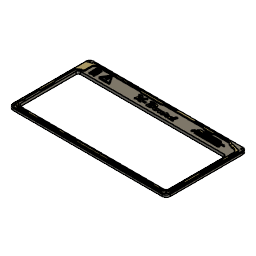
top (Autodesk Fusion 360 design; units mm, degrees)
part number: 2026-05-16-16-15-53-666
Autodesk Fusion 360 part; units mm, degrees
(part 1 of 5)
sketch "Sketch1" plane through (0, 0, 0) normal (0, 0, 1) x (1, 0, 0)
  line L0 (47.7197, -65.9177) -> (60.7197, -65.9177)
  line L1 (52.4822, -41.8177) -> (65.4822, -41.8177)
  line L2 (52.4822, -27.8177) -> (65.4822, -27.8177)
  arc A0 (170.2572, -3.7177) -> (170.7572, -3.2177) centre (170.2572, -3.2177) ccw
  line L3 (189.8072, 9.7823) -> (189.8072, -3.2177)
  arc A1 (180.2822, -9.2677) -> (179.7822, -8.7677) centre (179.7822, -9.2677) ccw
  line L4 (208.8572, 9.7823) -> (208.8572, -3.2177)
  arc A2 (208.8572, 9.7823) -> (208.3572, 10.2823) centre (208.3572, 9.7823) ccw
  arc A3 (195.3572, 10.2823) -> (194.8572, 9.7823) centre (195.3572, 9.7823) ccw
  arc A4 (182.2202, -9.7677) -> (181.7202, -10.2677) centre (182.2202, -10.2677) ccw
  arc A5 (208.3572, -3.7177) -> (208.8572, -3.2177) centre (208.3572, -3.2177) ccw
  line L5 (195.3572, 10.2823) -> (208.3572, 10.2823)
  line L6 (195.3572, -3.7177) -> (208.3572, -3.7177)
  line L7 (176.3072, -3.7177) -> (189.3072, -3.7177)
  line L8 (176.3072, 10.2823) -> (189.3072, 10.2823)
  arc A6 (175.8072, -3.2177) -> (176.3072, -3.7177) centre (176.3072, -3.2177) ccw
  arc A7 (195.3572, -8.7677) -> (194.8572, -9.2677) centre (195.3572, -9.2677) ccw
  arc A8 (176.3072, 10.2823) -> (175.8072, 9.7823) centre (176.3072, 9.7823) ccw
  line L9 (195.3572, -8.7677) -> (208.3572, -8.7677)
  arc A9 (170.7572, 9.7823) -> (170.2572, 10.2823) centre (170.2572, 9.7823) ccw
  arc A10 (177.9009, -47.3677) -> (177.4009, -46.8677) centre (177.4009, -47.3677) ccw
  arc A11 (208.8572, -28.3177) -> (208.3572, -27.8177) centre (208.3572, -28.3177) ccw
  arc A12 (171.5447, -27.8177) -> (171.0447, -28.3177) centre (171.5447, -28.3177) ccw
  line L10 (146.9447, -47.3677) -> (146.9447, -60.3677)
  arc A13 (188.2202, -24.7677) -> (188.7202, -24.2677) centre (188.2202, -24.2677) ccw
  line L11 (171.0447, -28.3177) -> (171.0447, -41.3177)
  line L12 (-5.4553, -47.3677) -> (-5.4553, -60.3677)
  arc A14 (195.3572, -27.8177) -> (194.8572, -28.3177) centre (195.3572, -28.3177) ccw
  arc A15 (162.4629, -48.3677) -> (161.9629, -47.8677) centre (161.9629, -48.3677) ccw
  line L13 (208.8572, -9.2677) -> (208.8572, -22.2677)
  line L14 (132.9447, -47.3677) -> (132.9447, -60.3677)
  arc A16 (195.3572, -46.8677) -> (194.8572, -47.3677) centre (195.3572, -47.3677) ccw
  line L15 (180.2822, -9.2677) -> (180.2822, -22.2677)
  arc A17 (186.3389, -48.3677) -> (185.8389, -47.8677) centre (185.8389, -48.3677) ccw
  line L16 (181.7202, -10.2677) -> (181.7202, -24.2677)
  line L17 (-24.5053, -47.3677) -> (-24.5053, -60.3677)
  line L18 (-113.7226, -118.8427) -> (-113.7226, 57.4273)
  line L19 (42.9572, 10.2823) -> (55.9572, 10.2823)
  line L20 (188.7202, -10.2677) -> (188.7202, -24.2677)
  arc A18 (37.4072, -9.2677) -> (36.9072, -8.7677) centre (36.9072, -9.2677) ccw
  line L21 (-43.5553, -47.3677) -> (-43.5553, -60.3677)
  line L22 (194.8572, -9.2677) -> (194.8572, -22.2677)
  line L23 (75.7947, -47.3677) -> (75.7947, -60.3677)
  line L24 (-57.5553, -47.3677) -> (-57.5553, -60.3677)
  line L25 (194.8572, -47.3677) -> (194.8572, -60.3677)
  line L26 (42.9572, -3.7177) -> (55.9572, -3.7177)
  line L27 (177.9009, -47.3677) -> (177.9009, -60.3677)
  arc A19 (55.9572, -3.7177) -> (56.4572, -3.2177) centre (55.9572, -3.2177) ccw
  arc A20 (56.4572, 9.7823) -> (55.9572, 10.2823) centre (55.9572, 9.7823) ccw
  arc A21 (17.8572, -3.7177) -> (18.3572, -3.2177) centre (17.8572, -3.2177) ccw
  line L28 (194.8572, 9.7823) -> (194.8572, -3.2177)
  arc A22 (194.8572, -3.2177) -> (195.3572, -3.7177) centre (195.3572, -3.2177) ccw
  line L29 (175.8072, 9.7823) -> (175.8072, -3.2177)
  arc A23 (188.7202, -10.2677) -> (188.2202, -9.7677) centre (188.2202, -10.2677) ccw
  arc A24 (208.8572, -47.3677) -> (208.3572, -46.8677) centre (208.3572, -47.3677) ccw
  line L30 (171.5447, -27.8177) -> (184.5447, -27.8177)
  arc A25 (179.7822, -22.7677) -> (180.2822, -22.2677) centre (179.7822, -22.2677) ccw
  line L31 (163.9009, -47.3677) -> (163.9009, -60.3677)
  line L32 (195.3572, -46.8677) -> (208.3572, -46.8677)
  line L33 (94.8447, -47.3677) -> (94.8447, -60.3677)
  line L34 (182.2202, -24.7677) -> (188.2202, -24.7677)
  line L35 (179.8389, -47.8677) -> (185.8389, -47.8677)
  line L36 (208.8572, -28.3177) -> (208.8572, -41.3177)
  arc A26 (184.5447, -41.8177) -> (185.0447, -41.3177) centre (184.5447, -41.3177) ccw
  arc A27 (185.0447, -28.3177) -> (184.5447, -27.8177) centre (184.5447, -28.3177) ccw
  arc A28 (189.3072, -3.7177) -> (189.8072, -3.2177) centre (189.3072, -3.2177) ccw
  arc A29 (189.8072, 9.7823) -> (189.3072, 10.2823) centre (189.3072, 9.7823) ccw
  line L37 (182.2202, -9.7677) -> (188.2202, -9.7677)
  line L38 (47.7197, -79.9177) -> (60.7197, -79.9177)
  line L39 (57.2447, -46.8677) -> (70.2447, -46.8677)
  line L40 (-113.7226, 57.4273) -> (228.9474, 57.4273)
  line L41 (18.6447, -47.3677) -> (18.6447, -60.3677)
  line L42 (89.7947, -47.3677) -> (89.7947, -60.3677)
  arc A30 (36.9072, -3.7177) -> (37.4072, -3.2177) centre (36.9072, -3.2177) ccw
  arc A31 (42.9572, -8.7677) -> (42.4572, -9.2677) centre (42.9572, -9.2677) ccw
  line L43 (56.7447, -47.3677) -> (56.7447, -60.3677)
  line L44 (51.6947, -47.3677) -> (51.6947, -60.3677)
  line L45 (-0.4053, -47.3677) -> (-0.4053, -60.3677)
  line L46 (208.8572, -47.3677) -> (208.8572, -60.3677)
  arc A32 (37.4072, 9.7823) -> (36.9072, 10.2823) centre (36.9072, 9.7823) ccw
  line L47 (13.5947, -47.3677) -> (13.5947, -60.3677)
  line L48 (-83.7491, -47.3677) -> (-83.7491, -60.3677)
  line L49 (-38.5053, -47.3677) -> (-38.5053, -60.3677)
  line L50 (127.8947, -47.3677) -> (127.8947, -60.3677)
  line L51 (37.6947, -47.3677) -> (37.6947, -60.3677)
  arc A33 (23.9072, -8.7677) -> (23.4072, -9.2677) centre (23.9072, -9.2677) ccw
  arc A34 (179.8389, -47.8677) -> (179.3389, -48.3677) centre (179.8389, -48.3677) ccw
  line L52 (70.7447, -47.3677) -> (70.7447, -60.3677)
  line L53 (-19.4553, -47.3677) -> (-19.4553, -60.3677)
  arc A35 (56.4572, -9.2677) -> (55.9572, -8.7677) centre (55.9572, -9.2677) ccw
  line L54 (113.8947, -47.3677) -> (113.8947, -60.3677)
  arc A36 (23.9072, 10.2823) -> (23.4072, 9.7823) centre (23.9072, 9.7823) ccw
  line L55 (108.8447, -47.3677) -> (108.8447, -60.3677)
  line L56 (-69.7491, -47.3677) -> (-69.7491, -60.3677)
  line L57 (32.6447, -47.3677) -> (32.6447, -60.3677)
  line L58 (-18.9553, -60.8677) -> (-5.9553, -60.8677)
  line L59 (-23.7178, -27.8177) -> (-10.7178, -27.8177)
  line L60 (228.9474, 57.4273) -> (228.9474, -118.8427)
  arc A37 (18.3572, -9.2677) -> (17.8572, -8.7677) centre (17.8572, -9.2677) ccw
  line L61 (-28.4803, -65.9177) -> (-15.4803, -65.9177)
  line L62 (-33.2428, 10.2823) -> (-20.2428, 10.2823)
  arc A38 (42.4572, -3.2177) -> (42.9572, -3.7177) centre (42.9572, -3.2177) ccw
  line L63 (23.9072, -8.7677) -> (36.9072, -8.7677)
  line L64 (-33.2428, -8.7677) -> (-20.2428, -8.7677)
  line L65 (42.4572, 9.7823) -> (42.4572, -3.2177)
  line L66 (-23.7178, -41.8177) -> (-10.7178, -41.8177)
  line L67 (18.3572, 9.7823) -> (18.3572, -3.2177)
  line L68 (119.1572, -8.7677) -> (132.1572, -8.7677)
  arc A39 (155.9629, -47.8677) -> (155.4629, -48.3677) centre (155.9629, -48.3677) ccw
  line L69 (-28.4803, -79.9177) -> (-15.4803, -79.9177)
  line L70 (123.9197, -79.9177) -> (136.9197, -79.9177)
  line L71 (-57.0553, -60.8677) -> (-44.0553, -60.8677)
  line L72 (128.6822, -27.8177) -> (141.6822, -27.8177)
  line L73 (-64.1991, -98.9677) -> (-51.1991, -98.9677)
  line L74 (-64.1991, -84.9677) -> (-51.1991, -84.9677)
  line L75 (128.6822, -41.8177) -> (141.6822, -41.8177)
  line L76 (42.9572, -8.7677) -> (55.9572, -8.7677)
  line L77 (9.6197, -79.9177) -> (22.6197, -79.9177)
  line L78 (19.1447, -60.8677) -> (32.1447, -60.8677)
  line L79 (-33.2428, -22.7677) -> (-20.2428, -22.7677)
  line L80 (133.4447, -60.8677) -> (146.4447, -60.8677)
  arc A40 (157.2572, 10.2823) -> (156.7572, 9.7823) centre (157.2572, 9.7823) ccw
  line L81 (123.9197, -65.9177) -> (136.9197, -65.9177)
  line L82 (9.6197, -65.9177) -> (22.6197, -65.9177)
  line L83 (119.1572, -22.7677) -> (132.1572, -22.7677)
  line L84 (119.1572, -3.7177) -> (132.1572, -3.7177)
  line L85 (28.6697, -79.9177) -> (41.6697, -79.9177)
  line L86 (119.1572, 10.2823) -> (132.1572, 10.2823)
  line L87 (85.8197, -65.9177) -> (98.8197, -65.9177)
  line L88 (37.4072, 9.7823) -> (37.4072, -3.2177)
  line L89 (138.2072, -8.7677) -> (151.2072, -8.7677)
  line L90 (4.8572, -8.7677) -> (17.8572, -8.7677)
  line L91 (-9.4303, -79.9177) -> (3.5697, -79.9177)
  line L92 (-9.9303, -66.4177) -> (-9.9303, -79.4177)
  arc A41 (-44.0553, -60.8677) -> (-43.5553, -60.3677) centre (-44.0553, -60.3677) ccw
  line L93 (-78.9866, -66.4177) -> (-78.9866, -79.4177)
  line L94 (-15.4491, -85.9677) -> (-9.4491, -85.9677)
  line L95 (-86.9246, -66.9177) -> (-80.9246, -66.9177)
  arc A42 (132.6572, -9.2677) -> (132.1572, -8.7677) centre (132.1572, -9.2677) ccw
  arc A43 (85.8197, -65.9177) -> (85.3197, -66.4177) centre (85.8197, -66.4177) ccw
  arc A44 (-64.6991, -98.4677) -> (-64.1991, -98.9677) centre (-64.1991, -98.4677) ccw
  arc A45 (28.1697, -79.4177) -> (28.6697, -79.9177) centre (28.6697, -79.4177) ccw
  arc A46 (-56.5486, -67.4177) -> (-57.0486, -66.9177) centre (-57.0486, -67.4177) ccw
  arc A47 (56.7447, -60.3677) -> (57.2447, -60.8677) centre (57.2447, -60.3677) ccw
  line L96 (-71.3428, 10.2823) -> (-58.3428, 10.2823)
  line L97 (-9.4303, -65.9177) -> (3.5697, -65.9177)
  arc A48 (156.7572, -3.2177) -> (157.2572, -3.7177) centre (157.2572, -3.2177) ccw
  line L98 (4.8572, 10.2823) -> (17.8572, 10.2823)
  line L99 (31.0509, -84.9677) -> (44.0509, -84.9677)
  line L100 (-88.0116, -98.9677) -> (-75.0116, -98.9677)
  arc A49 (32.1447, -60.8677) -> (32.6447, -60.3677) centre (32.1447, -60.3677) ccw
  arc A50 (44.5509, -85.4677) -> (44.0509, -84.9677) centre (44.0509, -85.4677) ccw
  line L101 (56.4572, 9.7823) -> (56.4572, -3.2177)
  arc A51 (189.3072, -79.9177) -> (189.8072, -79.4177) centre (189.3072, -79.4177) ccw
  arc A52 (-28.9803, -79.4177) -> (-28.4803, -79.9177) centre (-28.4803, -79.4177) ccw
  line L102 (28.1697, -66.4177) -> (28.1697, -79.4177)
  arc A53 (175.8072, -79.4177) -> (176.3072, -79.9177) centre (176.3072, -79.4177) ccw
  arc A54 (66.7697, -65.9177) -> (66.2697, -66.4177) centre (66.7697, -66.4177) ccw
  arc A55 (99.3197, -66.4177) -> (98.8197, -65.9177) centre (98.8197, -66.4177) ccw
  arc A56 (47.2197, -79.4177) -> (47.7197, -79.9177) centre (47.7197, -79.4177) ccw
  line L103 (23.4072, -9.2677) -> (23.4072, -22.2677)
  line L104 (-47.5303, -65.9177) -> (-34.5303, -65.9177)
  arc A57 (37.6947, -60.3677) -> (38.1947, -60.8677) centre (38.1947, -60.3677) ccw
  arc A58 (23.1197, -66.4177) -> (22.6197, -65.9177) centre (22.6197, -66.4177) ccw
  arc A59 (137.7072, -3.2177) -> (138.2072, -3.7177) centre (138.2072, -3.2177) ccw
  arc A60 (208.3572, -79.9177) -> (208.8572, -79.4177) centre (208.3572, -79.4177) ccw
  arc A61 (-63.0486, -66.9177) -> (-63.5486, -67.4177) centre (-63.0486, -67.4177) ccw
  line L105 (99.6072, -9.2677) -> (99.6072, -22.2677)
  line L106 (30.5509, -85.4677) -> (30.5509, -98.4677)
  arc A62 (194.8572, -79.4177) -> (195.3572, -79.9177) centre (195.3572, -79.4177) ccw
  arc A63 (31.0509, -84.9677) -> (30.5509, -85.4677) centre (31.0509, -85.4677) ccw
  arc A64 (-86.9246, -66.9177) -> (-87.4246, -67.4177) centre (-86.9246, -67.4177) ccw
  arc A65 (-14.9803, -66.4177) -> (-15.4803, -65.9177) centre (-15.4803, -66.4177) ccw
  line L107 (-28.9803, -66.4177) -> (-28.9803, -79.4177)
  line L108 (138.2072, -3.7177) -> (151.2072, -3.7177)
  line L109 (0.0947, -60.8677) -> (13.0947, -60.8677)
  arc A66 (-75.0116, -98.9677) -> (-74.5116, -98.4677) centre (-75.0116, -98.4677) ccw
  arc A67 (42.1697, -66.4177) -> (41.6697, -65.9177) centre (41.6697, -66.4177) ccw
  arc A68 (158.3442, -9.7677) -> (157.8442, -10.2677) centre (158.3442, -10.2677) ccw
  arc A69 (132.9447, -60.3677) -> (133.4447, -60.8677) centre (133.4447, -60.3677) ccw
  line L110 (-63.0486, -81.9177) -> (-57.0486, -81.9177)
  line L111 (-14.6928, -9.2677) -> (-14.6928, -22.2677)
  line L112 (-88.5116, -85.4677) -> (-88.5116, -98.4677)
  line L113 (164.4009, -46.8677) -> (177.4009, -46.8677)
  line L114 (-86.9246, -81.9177) -> (-80.9246, -81.9177)
  line L115 (23.1197, -66.4177) -> (23.1197, -79.4177)
  arc A70 (-0.4053, -60.3677) -> (0.0947, -60.8677) centre (0.0947, -60.3677) ccw
  arc A71 (98.8197, -79.9177) -> (99.3197, -79.4177) centre (98.8197, -79.4177) ccw
  line L116 (61.5072, -9.2677) -> (61.5072, -22.2677)
  line L117 (-64.6991, -85.4677) -> (-64.6991, -98.4677)
  arc A72 (-65.4866, -79.9177) -> (-64.9866, -79.4177) centre (-65.4866, -79.4177) ccw
  arc A73 (132.6572, 9.7823) -> (132.1572, 10.2823) centre (132.1572, 9.7823) ccw
  arc A74 (-27.3866, -98.9677) -> (-26.8866, -98.4677) centre (-27.3866, -98.4677) ccw
  arc A75 (47.7197, -65.9177) -> (47.2197, -66.4177) centre (47.7197, -66.4177) ccw
  arc A76 (138.2072, -8.7677) -> (137.7072, -9.2677) centre (138.2072, -9.2677) ccw
  arc A77 (18.3572, 9.7823) -> (17.8572, 10.2823) centre (17.8572, 9.7823) ccw
  arc A78 (28.6697, -65.9177) -> (28.1697, -66.4177) centre (28.6697, -66.4177) ccw
  line L118 (-71.3428, -8.7677) -> (-58.3428, -8.7677)
  line L119 (-71.3428, -3.7177) -> (-58.3428, -3.7177)
  arc A79 (42.9572, 10.2823) -> (42.4572, 9.7823) centre (42.9572, 9.7823) ccw
  line L120 (164.4009, -60.8677) -> (177.4009, -60.8677)
  line L121 (81.0572, 10.2823) -> (94.0572, 10.2823)
  line L122 (157.2572, -3.7177) -> (170.2572, -3.7177)
  line L123 (81.0572, -8.7677) -> (94.0572, -8.7677)
  line L124 (38.1947, -60.8677) -> (51.1947, -60.8677)
  arc A80 (132.1572, -3.7177) -> (132.6572, -3.2177) centre (132.1572, -3.2177) ccw
  arc A81 (-87.4246, -81.4177) -> (-86.9246, -81.9177) centre (-86.9246, -81.4177) ccw
  arc A82 (164.8442, -10.2677) -> (164.3442, -9.7677) centre (164.3442, -10.2677) ccw
  arc A83 (-8.9491, -86.4677) -> (-9.4491, -85.9677) centre (-9.4491, -86.4677) ccw
  arc A84 (13.0947, -60.8677) -> (13.5947, -60.3677) centre (13.0947, -60.3677) ccw
  line L125 (95.3447, -60.8677) -> (108.3447, -60.8677)
  line L126 (-38.0053, -60.8677) -> (-25.0053, -60.8677)
  arc A85 (-80.9246, -81.9177) -> (-80.4246, -81.4177) centre (-80.9246, -81.4177) ccw
  line L127 (90.5822, -27.8177) -> (103.5822, -27.8177)
  arc A86 (-57.0486, -81.9177) -> (-56.5486, -81.4177) centre (-57.0486, -81.4177) ccw
  line L128 (166.7822, -8.7677) -> (179.7822, -8.7677)
  line L129 (-33.2428, -3.7177) -> (-20.2428, -3.7177)
  line L130 (132.6572, 9.7823) -> (132.6572, -3.2177)
  line L131 (23.4072, 9.7823) -> (23.4072, -3.2177)
  line L132 (-61.8178, -27.8177) -> (-48.8178, -27.8177)
  line L133 (81.0572, -3.7177) -> (94.0572, -3.7177)
  line L134 (23.9072, -3.7177) -> (36.9072, -3.7177)
  arc A87 (41.6697, -79.9177) -> (42.1697, -79.4177) centre (41.6697, -79.4177) ccw
  line L135 (90.5822, -41.8177) -> (103.5822, -41.8177)
  arc A88 (-63.5486, -81.4177) -> (-63.0486, -81.9177) centre (-63.0486, -81.4177) ccw
  line L136 (-40.3866, -98.9677) -> (-27.3866, -98.9677)
  arc A89 (-25.0053, -60.8677) -> (-24.5053, -60.3677) centre (-25.0053, -60.3677) ccw
  line L137 (137.7072, 9.7823) -> (137.7072, -3.2177)
  line L138 (4.8572, -3.7177) -> (17.8572, -3.7177)
  line L139 (14.3822, -41.8177) -> (27.3822, -41.8177)
  line L140 (4.8572, -22.7677) -> (17.8572, -22.7677)
  arc A90 (23.4072, -3.2177) -> (23.9072, -3.7177) centre (23.9072, -3.2177) ccw
  line L141 (-47.5303, -79.9177) -> (-34.5303, -79.9177)
  line L142 (85.8197, -79.9177) -> (98.8197, -79.9177)
  line L143 (81.0572, -22.7677) -> (94.0572, -22.7677)
  line L144 (-56.5486, -67.4177) -> (-56.5486, -81.4177)
  arc A91 (-9.9303, -79.4177) -> (-9.4303, -79.9177) centre (-9.4303, -79.4177) ccw
  line L145 (23.9072, 10.2823) -> (36.9072, 10.2823)
  line L146 (-34.0303, -66.4177) -> (-34.0303, -79.4177)
  line L147 (14.3822, -27.8177) -> (27.3822, -27.8177)
  arc A92 (194.8572, -41.3177) -> (195.3572, -41.8177) centre (195.3572, -41.3177) ccw
  arc A93 (194.8572, -22.2677) -> (195.3572, -22.7677) centre (195.3572, -22.2677) ccw
  line L148 (194.8572, -28.3177) -> (194.8572, -41.3177)
  line L149 (195.3572, -22.7677) -> (208.3572, -22.7677)
  arc A94 (208.3572, -41.8177) -> (208.8572, -41.3177) centre (208.3572, -41.3177) ccw
  line L150 (185.0447, -28.3177) -> (185.0447, -41.3177)
  line L151 (195.3572, -41.8177) -> (208.3572, -41.8177)
  arc A95 (181.7202, -24.2677) -> (182.2202, -24.7677) centre (182.2202, -24.2677) ccw
  arc A96 (208.3572, -22.7677) -> (208.8572, -22.2677) centre (208.3572, -22.2677) ccw
  line L152 (171.5447, -41.8177) -> (184.5447, -41.8177)
  arc A97 (171.0447, -41.3177) -> (171.5447, -41.8177) centre (171.5447, -41.3177) ccw
  line L153 (195.3572, -27.8177) -> (208.3572, -27.8177)
  line L154 (57.2447, -60.8677) -> (70.2447, -60.8677)
  line L155 (228.9474, -118.8427) -> (-113.7226, -118.8427)
  line L156 (123.1322, -28.3177) -> (123.1322, -41.3177)
  arc A98 (114.3947, -46.8677) -> (113.8947, -47.3677) centre (114.3947, -47.3677) ccw
  line L157 (156.7572, -85.4677) -> (156.7572, -98.4677)
  line L158 (151.7072, -85.4677) -> (151.7072, -98.4677)
  arc A99 (-71.8428, -22.2677) -> (-71.3428, -22.7677) centre (-71.3428, -22.2677) ccw
  line L159 (-57.0553, -46.8677) -> (-44.0553, -46.8677)
  arc A100 (-69.7491, -47.3677) -> (-70.2491, -46.8677) centre (-70.2491, -47.3677) ccw
  arc A101 (-90.8928, -22.2677) -> (-90.3928, -22.7677) centre (-90.3928, -22.2677) ccw
  arc A102 (170.2572, -98.9677) -> (170.7572, -98.4677) centre (170.2572, -98.4677) ccw
  arc A103 (-86.1303, -41.3177) -> (-85.6303, -41.8177) centre (-85.6303, -41.3177) ccw
  arc A104 (149.6134, -79.4177) -> (150.1134, -79.9177) centre (150.1134, -79.4177) ccw
  arc A105 (-85.6303, -27.8177) -> (-86.1303, -28.3177) centre (-85.6303, -28.3177) ccw
  line L160 (8.8322, -28.3177) -> (8.8322, -41.3177)
  arc A106 (-77.3928, -22.7677) -> (-76.8928, -22.2677) centre (-77.3928, -22.2677) ccw
  line L161 (95.3447, -46.8677) -> (108.3447, -46.8677)
  line L162 (-29.2678, -28.3177) -> (-29.2678, -41.3177)
  arc A107 (-38.0053, -46.8677) -> (-38.5053, -47.3677) centre (-38.0053, -47.3677) ccw
  line L163 (-85.6303, -27.8177) -> (-72.6303, -27.8177)
  arc A108 (163.1134, -79.9177) -> (163.6134, -79.4177) centre (163.1134, -79.4177) ccw
  arc A109 (-33.7428, -22.2677) -> (-33.2428, -22.7677) centre (-33.2428, -22.2677) ccw
  line L164 (114.3947, -46.8677) -> (127.3947, -46.8677)
  arc A110 (14.3822, -27.8177) -> (13.8822, -28.3177) centre (14.3822, -28.3177) ccw
  arc A111 (-58.3428, -22.7677) -> (-57.8428, -22.2677) centre (-58.3428, -22.2677) ccw
  arc A112 (161.9629, -62.8677) -> (162.4629, -62.3677) centre (161.9629, -62.3677) ccw
  line L165 (-85.6303, -41.8177) -> (-72.6303, -41.8177)
  arc A113 (-42.7678, -27.8177) -> (-43.2678, -28.3177) centre (-42.7678, -28.3177) ccw
  arc A114 (163.9009, -60.3677) -> (164.4009, -60.8677) centre (164.4009, -60.3677) ccw
  line L166 (-18.9553, -46.8677) -> (-5.9553, -46.8677)
  arc A115 (-29.2678, -28.3177) -> (-29.7678, -27.8177) centre (-29.7678, -28.3177) ccw
  arc A116 (-4.6678, -27.8177) -> (-5.1678, -28.3177) centre (-4.6678, -28.3177) ccw
  line L167 (137.4197, -66.4177) -> (137.4197, -79.4177)
  line L168 (163.6134, -66.4177) -> (163.6134, -79.4177)
  arc A117 (-83.2491, -46.8677) -> (-83.7491, -47.3677) centre (-83.2491, -47.3677) ccw
  arc A118 (146.4447, -60.8677) -> (146.9447, -60.3677) centre (146.4447, -60.3677) ccw
  line L169 (170.7572, -85.4677) -> (170.7572, -98.4677)
  line L170 (157.2572, -84.9677) -> (170.2572, -84.9677)
  arc A119 (-39.2928, -22.7677) -> (-38.7928, -22.2677) centre (-39.2928, -22.2677) ccw
  arc A120 (-24.2178, -41.3177) -> (-23.7178, -41.8177) centre (-23.7178, -41.3177) ccw
  arc A121 (-29.7678, -41.8177) -> (-29.2678, -41.3177) centre (-29.7678, -41.3177) ccw
  arc A122 (-48.8178, -41.8177) -> (-48.3178, -41.3177) centre (-48.8178, -41.3177) ccw
  arc A123 (151.2072, -98.9677) -> (151.7072, -98.4677) centre (151.2072, -98.4677) ccw
  arc A124 (-43.5553, -47.3677) -> (-44.0553, -46.8677) centre (-44.0553, -47.3677) ccw
  arc A125 (208.8572, -9.2677) -> (208.3572, -8.7677) centre (208.3572, -9.2677) ccw
  line L171 (170.7572, 9.7823) -> (170.7572, -3.2177)
  arc A126 (-72.1303, -28.3177) -> (-72.6303, -27.8177) centre (-72.6303, -28.3177) ccw
  arc A127 (0.0947, -46.8677) -> (-0.4053, -47.3677) centre (0.0947, -47.3677) ccw
  arc A128 (122.6322, -41.8177) -> (123.1322, -41.3177) centre (122.6322, -41.3177) ccw
  line L172 (13.8822, -28.3177) -> (13.8822, -41.3177)
  line L173 (155.9629, -62.8677) -> (161.9629, -62.8677)
  line L174 (147.7322, -27.8177) -> (160.7322, -27.8177)
  arc A129 (-62.3178, -41.3177) -> (-61.8178, -41.8177) centre (-61.8178, -41.3177) ccw
  line L175 (147.2322, -28.3177) -> (147.2322, -41.3177)
  line L176 (71.5322, -27.8177) -> (84.5322, -27.8177)
  line L177 (133.4447, -46.8677) -> (146.4447, -46.8677)
  line L178 (0.0947, -46.8677) -> (13.0947, -46.8677)
  line L179 (158.3442, -24.7677) -> (164.3442, -24.7677)
  arc A130 (-90.3928, 10.2823) -> (-90.8928, 9.7823) centre (-90.3928, 9.7823) ccw
  line L180 (-90.8928, 9.7823) -> (-90.8928, -3.2177)
  line L181 (-10.2178, -28.3177) -> (-10.2178, -41.3177)
  line L182 (100.1072, -22.7677) -> (113.1072, -22.7677)
  arc A131 (89.7947, -47.3677) -> (89.2947, -46.8677) centre (89.2947, -47.3677) ccw
  line L183 (-90.3928, 10.2823) -> (-77.3928, 10.2823)
  line L184 (-62.3178, -28.3177) -> (-62.3178, -41.3177)
  arc A132 (118.6572, -22.2677) -> (119.1572, -22.7677) centre (119.1572, -22.2677) ccw
  arc A133 (109.1322, -41.3177) -> (109.6322, -41.8177) centre (109.6322, -41.3177) ccw
  arc A134 (123.1322, -28.3177) -> (122.6322, -27.8177) centre (122.6322, -28.3177) ccw
  line L185 (137.7072, -85.4677) -> (137.7072, -98.4677)
  arc A135 (-52.7928, -22.2677) -> (-52.2928, -22.7677) centre (-52.2928, -22.2677) ccw
  line L186 (61.2197, -66.4177) -> (61.2197, -79.4177)
  line L187 (-71.8428, 9.7823) -> (-71.8428, -3.2177)
  line L188 (147.7322, -41.8177) -> (160.7322, -41.8177)
  arc A136 (113.1072, -22.7677) -> (113.6072, -22.2677) centre (113.1072, -22.2677) ccw
  arc A137 (142.1822, -28.3177) -> (141.6822, -27.8177) centre (141.6822, -28.3177) ccw
  line L189 (-43.2678, -28.3177) -> (-43.2678, -41.3177)
  arc A138 (-76.8928, -9.2677) -> (-77.3928, -8.7677) centre (-77.3928, -9.2677) ccw
  arc A139 (-48.3178, -28.3177) -> (-48.8178, -27.8177) centre (-48.8178, -28.3177) ccw
  line L190 (-90.3928, -8.7677) -> (-77.3928, -8.7677)
  arc A140 (104.0822, -28.3177) -> (103.5822, -27.8177) centre (103.5822, -28.3177) ccw
  line L191 (-14.1928, -22.7677) -> (-1.1928, -22.7677)
  arc A141 (156.7572, -98.4677) -> (157.2572, -98.9677) centre (157.2572, -98.4677) ccw
  arc A142 (-43.2678, -41.3177) -> (-42.7678, -41.8177) centre (-42.7678, -41.3177) ccw
  arc A143 (-18.9553, -46.8677) -> (-19.4553, -47.3677) centre (-18.9553, -47.3677) ccw
  arc A144 (-23.7178, -27.8177) -> (-24.2178, -28.3177) centre (-23.7178, -28.3177) ccw
  line L192 (-42.7678, -27.8177) -> (-29.7678, -27.8177)
  line L193 (-90.3928, -3.7177) -> (-77.3928, -3.7177)
  arc A145 (-77.3928, -3.7177) -> (-76.8928, -3.2177) centre (-77.3928, -3.2177) ccw
  arc A146 (13.5947, -47.3677) -> (13.0947, -46.8677) centre (13.0947, -47.3677) ccw
  arc A147 (-90.3928, -8.7677) -> (-90.8928, -9.2677) centre (-90.3928, -9.2677) ccw
  arc A148 (141.6822, -41.8177) -> (142.1822, -41.3177) centre (141.6822, -41.3177) ccw
  arc A149 (-61.8178, -27.8177) -> (-62.3178, -28.3177) centre (-61.8178, -28.3177) ccw
  arc A150 (164.3442, -24.7677) -> (164.8442, -24.2677) centre (164.3442, -24.2677) ccw
  arc A151 (-14.6928, -22.2677) -> (-14.1928, -22.7677) centre (-14.1928, -22.2677) ccw
  arc A152 (94.0572, -22.7677) -> (94.5572, -22.2677) centre (94.0572, -22.2677) ccw
  arc A153 (-90.8928, -3.2177) -> (-90.3928, -3.7177) centre (-90.3928, -3.2177) ccw
  arc A154 (-71.3428, -8.7677) -> (-71.8428, -9.2677) centre (-71.3428, -9.2677) ccw
  line L194 (161.2322, -28.3177) -> (161.2322, -41.3177)
  arc A155 (-72.6303, -41.8177) -> (-72.1303, -41.3177) centre (-72.6303, -41.3177) ccw
  arc A156 (128.6822, -27.8177) -> (128.1822, -28.3177) centre (128.6822, -28.3177) ccw
  arc A157 (170.7572, -85.4677) -> (170.2572, -84.9677) centre (170.2572, -85.4677) ccw
  arc A158 (13.8822, -41.3177) -> (14.3822, -41.8177) centre (14.3822, -41.3177) ccw
  line L195 (109.6322, -27.8177) -> (122.6322, -27.8177)
  line L196 (104.0822, -28.3177) -> (104.0822, -41.3177)
  arc A159 (99.6072, -22.2677) -> (100.1072, -22.7677) centre (100.1072, -22.2677) ccw
  arc A160 (164.4009, -46.8677) -> (163.9009, -47.3677) centre (164.4009, -47.3677) ccw
  line L197 (-90.3928, -22.7677) -> (-77.3928, -22.7677)
  line L198 (-76.8928, 9.7823) -> (-76.8928, -3.2177)
  arc A161 (8.3322, -41.8177) -> (8.8322, -41.3177) centre (8.3322, -41.3177) ccw
  arc A162 (-71.3428, 10.2823) -> (-71.8428, 9.7823) centre (-71.3428, 9.7823) ccw
  line L199 (100.1072, 10.2823) -> (113.1072, 10.2823)
  arc A163 (81.0572, -8.7677) -> (80.5572, -9.2677) centre (81.0572, -9.2677) ccw
  arc A164 (189.3072, -98.9677) -> (189.8072, -98.4677) centre (189.3072, -98.4677) ccw
  line L200 (109.6322, -41.8177) -> (122.6322, -41.8177)
  line L201 (-52.2928, -3.7177) -> (-39.2928, -3.7177)
  line L202 (176.3072, -84.9677) -> (189.3072, -84.9677)
  arc A165 (-19.7428, -9.2677) -> (-20.2428, -8.7677) centre (-20.2428, -9.2677) ccw
  arc A166 (33.4322, -27.8177) -> (32.9322, -28.3177) centre (33.4322, -28.3177) ccw
  line L203 (94.5572, 9.7823) -> (94.5572, -3.2177)
  line L204 (119.1572, -98.9677) -> (132.1572, -98.9677)
  line L205 (-71.3428, -22.7677) -> (-58.3428, -22.7677)
  arc A167 (113.1072, -98.9677) -> (113.6072, -98.4677) centre (113.1072, -98.4677) ccw
  line L206 (42.9572, -22.7677) -> (55.9572, -22.7677)
  arc A168 (62.0072, -8.7677) -> (61.5072, -9.2677) centre (62.0072, -9.2677) ccw
  arc A169 (4.3572, -22.2677) -> (4.8572, -22.7677) centre (4.8572, -22.2677) ccw
  line L207 (132.6572, -9.2677) -> (132.6572, -22.2677)
  line L208 (-38.7928, 9.7823) -> (-38.7928, -3.2177)
  arc A170 (84.0509, -100.4677) -> (84.5509, -100.9677) centre (84.5509, -100.4677) ccw
  line L209 (166.2822, -9.2677) -> (166.2822, -22.2677)
  line L210 (76.2947, -46.8677) -> (89.2947, -46.8677)
  line L211 (194.8572, -66.4177) -> (194.8572, -79.4177)
  arc A171 (85.0322, -28.3177) -> (84.5322, -27.8177) centre (84.5322, -28.3177) ccw
  line L212 (51.9822, -28.3177) -> (51.9822, -41.3177)
  arc A172 (71.0322, -41.3177) -> (71.5322, -41.8177) centre (71.5322, -41.3177) ccw
  arc A173 (89.2947, -60.8677) -> (89.7947, -60.3677) centre (89.2947, -60.3677) ccw
  arc A174 (189.8072, -66.4177) -> (189.3072, -65.9177) centre (189.3072, -66.4177) ccw
  line L213 (23.9072, -22.7677) -> (36.9072, -22.7677)
  arc A175 (-19.7428, 9.7823) -> (-20.2428, 10.2823) centre (-20.2428, 9.7823) ccw
  line L214 (132.6572, -85.4677) -> (132.6572, -98.4677)
  line L215 (189.8072, -85.4677) -> (189.8072, -98.4677)
  line L216 (100.1072, -84.9677) -> (113.1072, -84.9677)
  arc A176 (79.7697, -79.9177) -> (80.2697, -79.4177) centre (79.7697, -79.4177) ccw
  line L217 (-52.2928, 10.2823) -> (-39.2928, 10.2823)
  arc A177 (61.5072, -22.2677) -> (62.0072, -22.7677) centre (62.0072, -22.2677) ccw
  line L218 (162.4629, -48.3677) -> (162.4629, -62.3677)
  line L219 (-14.1928, -3.7177) -> (-1.1928, -3.7177)
  line L220 (155.9629, -47.8677) -> (161.9629, -47.8677)
  line L221 (100.1072, -98.9677) -> (113.1072, -98.9677)
  line L222 (-4.6678, -41.8177) -> (8.3322, -41.8177)
  line L223 (138.2072, -98.9677) -> (151.2072, -98.9677)
  arc A178 (4.3572, -3.2177) -> (4.8572, -3.7177) centre (4.8572, -3.2177) ccw
  arc A179 (75.5072, 9.7823) -> (75.0072, 10.2823) centre (75.0072, 9.7823) ccw
  arc A180 (113.6072, -85.4677) -> (113.1072, -84.9677) centre (113.1072, -85.4677) ccw
  arc A181 (27.8822, -28.3177) -> (27.3822, -27.8177) centre (27.3822, -28.3177) ccw
  line L224 (76.2947, -60.8677) -> (89.2947, -60.8677)
  arc A182 (70.2447, -60.8677) -> (70.7447, -60.3677) centre (70.2447, -60.3677) ccw
  arc A183 (55.9572, -22.7677) -> (56.4572, -22.2677) centre (55.9572, -22.2677) ccw
  line L225 (-57.8428, 9.7823) -> (-57.8428, -3.2177)
  arc A184 (80.2697, -66.4177) -> (79.7697, -65.9177) centre (79.7697, -66.4177) ccw
  arc A185 (-14.6928, -3.2177) -> (-14.1928, -3.7177) centre (-14.1928, -3.2177) ccw
  line L226 (208.8572, -66.4177) -> (208.8572, -79.4177)
  line L227 (-33.7428, 9.7823) -> (-33.7428, -3.2177)
  arc A186 (90.0822, -41.3177) -> (90.5822, -41.8177) centre (90.5822, -41.3177) ccw
  arc A187 (132.1572, -22.7677) -> (132.6572, -22.2677) centre (132.1572, -22.2677) ccw
  arc A188 (95.3447, -46.8677) -> (94.8447, -47.3677) centre (95.3447, -47.3677) ccw
  line L228 (62.0072, -3.7177) -> (75.0072, -3.7177)
  line L229 (66.7697, -65.9177) -> (79.7697, -65.9177)
  line L230 (118.6572, -85.4677) -> (118.6572, -98.4677)
  line L231 (157.8442, -10.2677) -> (157.8442, -24.2677)
  line L232 (-38.7928, -9.2677) -> (-38.7928, -22.2677)
  arc A189 (-1.1928, -3.7177) -> (-0.6928, -3.2177) centre (-1.1928, -3.2177) ccw
  arc A190 (118.6572, -98.4677) -> (119.1572, -98.9677) centre (119.1572, -98.4677) ccw
  line L233 (149.6134, -66.4177) -> (149.6134, -79.4177)
  line L234 (-76.8928, -9.2677) -> (-76.8928, -22.2677)
  arc A191 (161.2322, -28.3177) -> (160.7322, -27.8177) centre (160.7322, -28.3177) ccw
  arc A192 (103.5822, -41.8177) -> (104.0822, -41.3177) centre (103.5822, -41.3177) ccw
  line L235 (61.5072, 9.7823) -> (61.5072, -3.2177)
  arc A193 (80.5572, -3.2177) -> (81.0572, -3.7177) centre (81.0572, -3.2177) ccw
  line L236 (-33.7428, -9.2677) -> (-33.7428, -22.2677)
  arc A194 (195.3572, -65.9177) -> (194.8572, -66.4177) centre (195.3572, -66.4177) ccw
  line L237 (138.2072, -22.7677) -> (151.2072, -22.7677)
  arc A195 (-33.2428, -8.7677) -> (-33.7428, -9.2677) centre (-33.2428, -9.2677) ccw
  line L238 (113.6072, -85.4677) -> (113.6072, -98.4677)
  line L239 (-52.7928, -9.2677) -> (-52.7928, -22.2677)
  arc A196 (70.7447, -47.3677) -> (70.2447, -46.8677) centre (70.2447, -47.3677) ccw
  arc A197 (-38.7928, -9.2677) -> (-39.2928, -8.7677) centre (-39.2928, -9.2677) ccw
  line L240 (80.2697, -66.4177) -> (80.2697, -79.4177)
  line L241 (151.7072, -9.2677) -> (151.7072, -22.2677)
  arc A198 (-10.7178, -41.8177) -> (-10.2178, -41.3177) centre (-10.7178, -41.3177) ccw
  line L242 (-57.8428, -9.2677) -> (-57.8428, -22.2677)
  line L243 (71.0322, -28.3177) -> (71.0322, -41.3177)
  line L244 (195.3572, -65.9177) -> (208.3572, -65.9177)
  line L245 (65.9822, -28.3177) -> (65.9822, -41.3177)
  arc A199 (94.8447, -60.3677) -> (95.3447, -60.8677) centre (95.3447, -60.3677) ccw
  line L246 (62.0072, -8.7677) -> (75.0072, -8.7677)
  line L247 (-19.7428, 9.7823) -> (-19.7428, -3.2177)
  line L248 (-14.1928, -8.7677) -> (-1.1928, -8.7677)
  arc A200 (132.6572, -85.4677) -> (132.1572, -84.9677) centre (132.1572, -85.4677) ccw
  line L249 (-90.8928, -9.2677) -> (-90.8928, -22.2677)
  line L250 (138.2072, -84.9677) -> (151.2072, -84.9677)
  line L251 (62.0072, -22.7677) -> (75.0072, -22.7677)
  arc A201 (4.8572, 10.2823) -> (4.3572, 9.7823) centre (4.8572, 9.7823) ccw
  line L252 (-4.6678, -27.8177) -> (8.3322, -27.8177)
  arc A202 (147.2322, -41.3177) -> (147.7322, -41.8177) centre (147.7322, -41.3177) ccw
  line L253 (150.1134, -79.9177) -> (163.1134, -79.9177)
  arc A203 (128.1822, -41.3177) -> (128.6822, -41.8177) centre (128.6822, -41.3177) ccw
  arc A204 (166.2822, -22.2677) -> (166.7822, -22.7677) centre (166.7822, -22.2677) ccw
  arc A205 (137.4197, -66.4177) -> (136.9197, -65.9177) centre (136.9197, -66.4177) ccw
  arc A206 (-57.0553, -46.8677) -> (-57.5553, -47.3677) centre (-57.0553, -47.3677) ccw
  arc A207 (91.0509, -86.4677) -> (90.5509, -85.9677) centre (90.5509, -86.4677) ccw
  arc A208 (76.2947, -46.8677) -> (75.7947, -47.3677) centre (76.2947, -47.3677) ccw
  arc A209 (108.8447, -47.3677) -> (108.3447, -46.8677) centre (108.3447, -47.3677) ccw
  line L254 (85.0322, -28.3177) -> (85.0322, -41.3177)
  line L255 (84.0509, -86.4677) -> (84.0509, -100.4677)
  arc A210 (137.7072, -22.2677) -> (138.2072, -22.7677) centre (138.2072, -22.2677) ccw
  arc A211 (-5.4553, -47.3677) -> (-5.9553, -46.8677) centre (-5.9553, -47.3677) ccw
  arc A212 (-57.8428, 9.7823) -> (-58.3428, 10.2823) centre (-58.3428, 9.7823) ccw
  line L256 (66.2697, -66.4177) -> (66.2697, -79.4177)
  arc A213 (-52.7928, -3.2177) -> (-52.2928, -3.7177) centre (-52.2928, -3.2177) ccw
  arc A214 (138.2072, -84.9677) -> (137.7072, -85.4677) centre (138.2072, -85.4677) ccw
  line L257 (84.5509, -85.9677) -> (90.5509, -85.9677)
  arc A215 (8.8322, -28.3177) -> (8.3322, -27.8177) centre (8.3322, -28.3177) ccw
  line L258 (164.8442, -10.2677) -> (164.8442, -24.2677)
  line L259 (-38.0053, -46.8677) -> (-25.0053, -46.8677)
  arc A216 (127.8947, -47.3677) -> (127.3947, -46.8677) centre (127.3947, -47.3677) ccw
  arc A217 (194.8572, -60.3677) -> (195.3572, -60.8677) centre (195.3572, -60.3677) ccw
  line L260 (104.8697, -79.9177) -> (117.8697, -79.9177)
  line L261 (119.1572, -84.9677) -> (132.1572, -84.9677)
  arc A218 (-38.7928, 9.7823) -> (-39.2928, 10.2823) centre (-39.2928, 9.7823) ccw
  line L262 (71.5322, -41.8177) -> (84.5322, -41.8177)
  line L263 (-71.8428, -9.2677) -> (-71.8428, -22.2677)
  arc A219 (100.1072, -84.9677) -> (99.6072, -85.4677) centre (100.1072, -85.4677) ccw
  line L264 (-52.2928, -22.7677) -> (-39.2928, -22.7677)
  arc A220 (208.8572, -66.4177) -> (208.3572, -65.9177) centre (208.3572, -66.4177) ccw
  arc A221 (147.7322, -27.8177) -> (147.2322, -28.3177) centre (147.7322, -28.3177) ccw
  arc A222 (61.2197, -66.4177) -> (60.7197, -65.9177) centre (60.7197, -66.4177) ccw
  arc A223 (65.4822, -41.8177) -> (65.9822, -41.3177) centre (65.4822, -41.3177) ccw
  arc A224 (99.6072, -98.4677) -> (100.1072, -98.9677) centre (100.1072, -98.4677) ccw
  arc A225 (119.1572, -84.9677) -> (118.6572, -85.4677) centre (119.1572, -85.4677) ccw
  line L265 (142.1822, -28.3177) -> (142.1822, -41.3177)
  arc A226 (-5.1678, -41.3177) -> (-4.6678, -41.8177) centre (-4.6678, -41.3177) ccw
  arc A227 (150.1134, -65.9177) -> (149.6134, -66.4177) centre (150.1134, -66.4177) ccw
  arc A228 (151.2072, -22.7677) -> (151.7072, -22.2677) centre (151.2072, -22.2677) ccw
  arc A229 (-71.8428, -3.2177) -> (-71.3428, -3.7177) centre (-71.3428, -3.2177) ccw
  arc A230 (157.8442, -24.2677) -> (158.3442, -24.7677) centre (158.3442, -24.2677) ccw
  arc A231 (146.9447, -47.3677) -> (146.4447, -46.8677) centre (146.4447, -47.3677) ccw
  arc A232 (-1.1928, -22.7677) -> (-0.6928, -22.2677) centre (-1.1928, -22.2677) ccw
  line L266 (-72.1303, -28.3177) -> (-72.1303, -41.3177)
  line L267 (128.1822, -28.3177) -> (128.1822, -41.3177)
  arc A233 (-10.2178, -28.3177) -> (-10.7178, -27.8177) centre (-10.7178, -28.3177) ccw
  line L268 (109.1322, -28.3177) -> (109.1322, -41.3177)
  line L269 (-83.2491, -46.8677) -> (-70.2491, -46.8677)
  arc A234 (109.6322, -27.8177) -> (109.1322, -28.3177) centre (109.6322, -28.3177) ccw
  arc A235 (160.7322, -41.8177) -> (161.2322, -41.3177) centre (160.7322, -41.3177) ccw
  line L270 (-86.1303, -28.3177) -> (-86.1303, -41.3177)
  arc A236 (71.5322, -27.8177) -> (71.0322, -28.3177) centre (71.5322, -28.3177) ccw
  arc A237 (90.5509, -100.9677) -> (91.0509, -100.4677) centre (90.5509, -100.4677) ccw
  arc A238 (-20.2428, -22.7677) -> (-19.7428, -22.2677) centre (-20.2428, -22.2677) ccw
  arc A239 (84.5322, -41.8177) -> (85.0322, -41.3177) centre (84.5322, -41.3177) ccw
  line L271 (-5.1678, -28.3177) -> (-5.1678, -41.3177)
  line L272 (-42.7678, -41.8177) -> (-29.7678, -41.8177)
  arc A240 (-76.8928, 9.7823) -> (-77.3928, 10.2823) centre (-77.3928, 9.7823) ccw
  line L273 (155.4629, -48.3677) -> (155.4629, -62.3677)
  arc A241 (-24.5053, -47.3677) -> (-25.0053, -46.8677) centre (-25.0053, -47.3677) ccw
  line L274 (-48.3178, -28.3177) -> (-48.3178, -41.3177)
  arc A242 (133.4447, -46.8677) -> (132.9447, -47.3677) centre (133.4447, -47.3677) ccw
  line L275 (-24.2178, -28.3177) -> (-24.2178, -41.3177)
  arc A243 (18.6447, -60.3677) -> (19.1447, -60.8677) centre (19.1447, -60.3677) ccw
  arc A244 (177.4009, -60.8677) -> (177.9009, -60.3677) centre (177.4009, -60.3677) ccw
  line L276 (75.5072, 9.7823) -> (75.5072, -3.2177)
  arc A245 (-33.7428, -3.2177) -> (-33.2428, -3.7177) centre (-33.2428, -3.2177) ccw
  line L277 (-0.6928, -9.2677) -> (-0.6928, -22.2677)
  line L278 (91.0509, -86.4677) -> (91.0509, -100.4677)
  arc A246 (32.9322, -41.3177) -> (33.4322, -41.8177) centre (33.4322, -41.3177) ccw
  line L279 (195.3572, -84.9677) -> (208.3572, -84.9677)
  line L280 (195.3572, -79.9177) -> (208.3572, -79.9177)
  arc A247 (151.7072, -9.2677) -> (151.2072, -8.7677) centre (151.2072, -9.2677) ccw
  line L281 (-78.4866, -79.9177) -> (-65.4866, -79.9177)
  arc A248 (138.2072, 10.2823) -> (137.7072, 9.7823) centre (138.2072, 9.7823) ccw
  arc A249 (175.8072, -98.4677) -> (176.3072, -98.9677) centre (176.3072, -98.4677) ccw
  arc A250 (94.0572, -3.7177) -> (94.5572, -3.2177) centre (94.0572, -3.2177) ccw
  arc A251 (104.8697, -65.9177) -> (104.3697, -66.4177) centre (104.8697, -66.4177) ccw
  arc A252 (-0.6928, -9.2677) -> (-1.1928, -8.7677) centre (-1.1928, -9.2677) ccw
  arc A253 (163.6134, -66.4177) -> (163.1134, -65.9177) centre (163.1134, -66.4177) ccw
  line L282 (-40.3866, -84.9677) -> (-27.3866, -84.9677)
  line L283 (9.1197, -66.4177) -> (9.1197, -79.4177)
  line L284 (118.6572, 9.7823) -> (118.6572, -3.2177)
  line L285 (179.3389, -48.3677) -> (179.3389, -62.3677)
  line L286 (32.9322, -28.3177) -> (32.9322, -41.3177)
  line L287 (208.8572, -85.4677) -> (208.8572, -98.4677)
  line L288 (-14.9803, -66.4177) -> (-14.9803, -79.4177)
  arc A254 (137.7072, -98.4677) -> (138.2072, -98.9677) centre (138.2072, -98.4677) ccw
  line L289 (189.8072, -66.4177) -> (189.8072, -79.4177)
  line L290 (123.4197, -66.4177) -> (123.4197, -79.4177)
  arc A255 (104.3697, -79.4177) -> (104.8697, -79.9177) centre (104.8697, -79.4177) ccw
  arc A256 (36.9072, -22.7677) -> (37.4072, -22.2677) centre (36.9072, -22.2677) ccw
  line L291 (-52.7928, 9.7823) -> (-52.7928, -3.2177)
  line L292 (42.4572, -9.2677) -> (42.4572, -22.2677)
  arc A257 (90.5822, -27.8177) -> (90.0822, -28.3177) centre (90.5822, -28.3177) ccw
  arc A258 (208.3572, -98.9677) -> (208.8572, -98.4677) centre (208.3572, -98.4677) ccw
  arc A259 (151.7072, -85.4677) -> (151.2072, -84.9677) centre (151.2072, -85.4677) ccw
  arc A260 (166.7822, -8.7677) -> (166.2822, -9.2677) centre (166.7822, -9.2677) ccw
  arc A261 (-9.4491, -100.9677) -> (-8.9491, -100.4677) centre (-9.4491, -100.4677) ccw
  arc A262 (-26.8866, -85.4677) -> (-27.3866, -84.9677) centre (-27.3866, -85.4677) ccw
  line L293 (19.1447, -46.8677) -> (32.1447, -46.8677)
  line L294 (104.8697, -65.9177) -> (117.8697, -65.9177)
  arc A263 (-78.9866, -79.4177) -> (-78.4866, -79.9177) centre (-78.4866, -79.4177) ccw
  line L295 (33.4322, -41.8177) -> (46.4322, -41.8177)
  arc A264 (208.3572, -60.8677) -> (208.8572, -60.3677) centre (208.3572, -60.3677) ccw
  line L296 (-78.4866, -65.9177) -> (-65.4866, -65.9177)
  arc A265 (-50.6991, -85.4677) -> (-51.1991, -84.9677) centre (-51.1991, -85.4677) ccw
  arc A266 (27.3822, -41.8177) -> (27.8822, -41.3177) centre (27.3822, -41.3177) ccw
  arc A267 (113.6072, -9.2677) -> (113.1072, -8.7677) centre (113.1072, -9.2677) ccw
  arc A268 (-48.0303, -79.4177) -> (-47.5303, -79.9177) centre (-47.5303, -79.4177) ccw
  line L297 (46.9322, -28.3177) -> (46.9322, -41.3177)
  arc A269 (-20.2428, -3.7177) -> (-19.7428, -3.2177) centre (-20.2428, -3.2177) ccw
  line L298 (4.0697, -66.4177) -> (4.0697, -79.4177)
  arc A270 (75.7947, -60.3677) -> (76.2947, -60.8677) centre (76.2947, -60.3677) ccw
  arc A271 (4.0697, -66.4177) -> (3.5697, -65.9177) centre (3.5697, -66.4177) ccw
  arc A272 (194.8572, -98.4677) -> (195.3572, -98.9677) centre (195.3572, -98.4677) ccw
  line L299 (80.5572, 9.7823) -> (80.5572, -3.2177)
  line L300 (4.3572, 9.7823) -> (4.3572, -3.2177)
  line L301 (27.8822, -28.3177) -> (27.8822, -41.3177)
  line L302 (-63.0486, -66.9177) -> (-57.0486, -66.9177)
  arc A273 (61.5072, -3.2177) -> (62.0072, -3.7177) centre (62.0072, -3.2177) ccw
  arc A274 (-51.1991, -98.9677) -> (-50.6991, -98.4677) centre (-51.1991, -98.4677) ccw
  line L303 (-8.9491, -86.4677) -> (-8.9491, -100.4677)
  line L304 (175.8072, -66.4177) -> (175.8072, -79.4177)
  arc A275 (84.5509, -85.9677) -> (84.0509, -86.4677) centre (84.5509, -86.4677) ccw
  arc A276 (94.5572, -9.2677) -> (94.0572, -8.7677) centre (94.0572, -9.2677) ccw
  line L305 (166.7822, -22.7677) -> (179.7822, -22.7677)
  line L306 (176.3072, -98.9677) -> (189.3072, -98.9677)
  line L307 (66.7697, -79.9177) -> (79.7697, -79.9177)
  line L308 (195.3572, -60.8677) -> (208.3572, -60.8677)
  arc A277 (-14.1928, 10.2823) -> (-14.6928, 9.7823) centre (-14.1928, 9.7823) ccw
  arc A278 (100.1072, 10.2823) -> (99.6072, 9.7823) centre (100.1072, 9.7823) ccw
  arc A279 (81.0572, 10.2823) -> (80.5572, 9.7823) centre (81.0572, 9.7823) ccw
  line L309 (-0.6928, 9.7823) -> (-0.6928, -3.2177)
  line L310 (137.7072, -9.2677) -> (137.7072, -22.2677)
  line L311 (157.2572, -98.9677) -> (170.2572, -98.9677)
  line L312 (179.8389, -62.8677) -> (185.8389, -62.8677)
  arc A280 (62.0072, 10.2823) -> (61.5072, 9.7823) centre (62.0072, 9.7823) ccw
  arc A281 (-78.4866, -65.9177) -> (-78.9866, -66.4177) centre (-78.4866, -66.4177) ccw
  line L313 (33.4322, -27.8177) -> (46.4322, -27.8177)
  arc A282 (-19.4553, -60.3677) -> (-18.9553, -60.8677) centre (-18.9553, -60.3677) ccw
  arc A283 (9.6197, -65.9177) -> (9.1197, -66.4177) centre (9.6197, -66.4177) ccw
  line L314 (84.5509, -100.9677) -> (90.5509, -100.9677)
  line L315 (-83.2491, -60.8677) -> (-70.2491, -60.8677)
  arc A284 (119.1572, 10.2823) -> (118.6572, 9.7823) centre (119.1572, 9.7823) ccw
  arc A285 (-47.5303, -65.9177) -> (-48.0303, -66.4177) centre (-47.5303, -66.4177) ccw
  arc A286 (23.4072, -22.2677) -> (23.9072, -22.7677) centre (23.9072, -22.2677) ccw
  arc A287 (127.3947, -60.8677) -> (127.8947, -60.3677) centre (127.3947, -60.3677) ccw
  line L316 (118.6572, -9.2677) -> (118.6572, -22.2677)
  line L317 (62.0072, 10.2823) -> (75.0072, 10.2823)
  line L318 (175.8072, -85.4677) -> (175.8072, -98.4677)
  line L319 (-14.6928, 9.7823) -> (-14.6928, -3.2177)
  arc A288 (113.8947, -60.3677) -> (114.3947, -60.8677) centre (114.3947, -60.3677) ccw
  arc A289 (32.6447, -47.3677) -> (32.1447, -46.8677) centre (32.1447, -47.3677) ccw
  arc A290 (185.8389, -62.8677) -> (186.3389, -62.3677) centre (185.8389, -62.3677) ccw
  line L320 (90.0822, -28.3177) -> (90.0822, -41.3177)
  line L321 (99.6072, -85.4677) -> (99.6072, -98.4677)
  line L322 (195.3572, -98.9677) -> (208.3572, -98.9677)
  line L323 (-52.2928, -8.7677) -> (-39.2928, -8.7677)
  arc A291 (80.5572, -22.2677) -> (81.0572, -22.7677) centre (81.0572, -22.2677) ccw
  line L324 (-14.1928, 10.2823) -> (-1.1928, 10.2823)
  arc A292 (113.6072, 9.7823) -> (113.1072, 10.2823) centre (113.1072, 9.7823) ccw
  arc A293 (38.1947, -46.8677) -> (37.6947, -47.3677) centre (38.1947, -47.3677) ccw
  arc A294 (-40.3866, -84.9677) -> (-40.8866, -85.4677) centre (-40.3866, -85.4677) ccw
  line L325 (85.3197, -66.4177) -> (85.3197, -79.4177)
  arc A295 (132.1572, -98.9677) -> (132.6572, -98.4677) centre (132.1572, -98.4677) ccw
  arc A296 (46.4322, -41.8177) -> (46.9322, -41.3177) centre (46.4322, -41.3177) ccw
  line L326 (150.1134, -65.9177) -> (163.1134, -65.9177)
  line L327 (176.3072, -79.9177) -> (189.3072, -79.9177)
  line L328 (113.6072, -9.2677) -> (113.6072, -22.2677)
  arc A297 (-57.5553, -60.3677) -> (-57.0553, -60.8677) centre (-57.0553, -60.3677) ccw
  arc A298 (75.0072, -22.7677) -> (75.5072, -22.2677) centre (75.0072, -22.2677) ccw
  arc A299 (52.4822, -27.8177) -> (51.9822, -28.3177) centre (52.4822, -28.3177) ccw
  arc A300 (179.3389, -62.3677) -> (179.8389, -62.8677) centre (179.8389, -62.3677) ccw
  arc A301 (113.1072, -3.7177) -> (113.6072, -3.2177) centre (113.1072, -3.2177) ccw
  arc A302 (-38.5053, -60.3677) -> (-38.0053, -60.8677) centre (-38.0053, -60.3677) ccw
  arc A303 (157.2572, -84.9677) -> (156.7572, -85.4677) centre (157.2572, -85.4677) ccw
  arc A304 (94.5572, 9.7823) -> (94.0572, 10.2823) centre (94.0572, 9.7823) ccw
  arc A305 (46.9322, -28.3177) -> (46.4322, -27.8177) centre (46.4322, -28.3177) ccw
  arc A306 (-52.2928, 10.2823) -> (-52.7928, 9.7823) centre (-52.2928, 9.7823) ccw
  arc A307 (-70.2491, -60.8677) -> (-69.7491, -60.3677) centre (-70.2491, -60.3677) ccw
  arc A308 (-14.1928, -8.7677) -> (-14.6928, -9.2677) centre (-14.1928, -9.2677) ccw
  arc A309 (189.8072, -85.4677) -> (189.3072, -84.9677) centre (189.3072, -85.4677) ccw
  arc A310 (-34.5303, -79.9177) -> (-34.0303, -79.4177) centre (-34.5303, -79.4177) ccw
  arc A311 (75.5072, -9.2677) -> (75.0072, -8.7677) centre (75.0072, -9.2677) ccw
  line L329 (113.6072, 9.7823) -> (113.6072, -3.2177)
  arc A312 (-0.6928, 9.7823) -> (-1.1928, 10.2823) centre (-1.1928, 9.7823) ccw
  arc A313 (208.8572, -85.4677) -> (208.3572, -84.9677) centre (208.3572, -85.4677) ccw
  arc A314 (136.9197, -79.9177) -> (137.4197, -79.4177) centre (136.9197, -79.4177) ccw
  arc A315 (65.9822, -28.3177) -> (65.4822, -27.8177) centre (65.4822, -28.3177) ccw
  arc A316 (75.0072, -3.7177) -> (75.5072, -3.2177) centre (75.0072, -3.2177) ccw
  arc A317 (-15.9491, -100.4677) -> (-15.4491, -100.9677) centre (-15.4491, -100.4677) ccw
  line L330 (114.3947, -60.8677) -> (127.3947, -60.8677)
  arc A318 (195.3572, -84.9677) -> (194.8572, -85.4677) centre (195.3572, -85.4677) ccw
  arc A319 (123.4197, -79.4177) -> (123.9197, -79.9177) centre (123.9197, -79.4177) ccw
  arc A320 (-9.4303, -65.9177) -> (-9.9303, -66.4177) centre (-9.4303, -66.4177) ccw
  line L331 (94.5572, -9.2677) -> (94.5572, -22.2677)
  line L332 (4.3572, -9.2677) -> (4.3572, -22.2677)
  line L333 (-74.5116, -85.4677) -> (-74.5116, -98.4677)
  arc A321 (30.5509, -98.4677) -> (31.0509, -98.9677) centre (31.0509, -98.4677) ccw
  arc A322 (42.4572, -22.2677) -> (42.9572, -22.7677) centre (42.9572, -22.2677) ccw
  arc A323 (-15.4491, -85.9677) -> (-15.9491, -86.4677) centre (-15.4491, -86.4677) ccw
  line L334 (-61.8178, -41.8177) -> (-48.8178, -41.8177)
  line L335 (158.3442, -9.7677) -> (164.3442, -9.7677)
  line L336 (-63.5486, -67.4177) -> (-63.5486, -81.4177)
  line L337 (194.8572, -85.4677) -> (194.8572, -98.4677)
  line L338 (42.1697, -66.4177) -> (42.1697, -79.4177)
  line L339 (99.6072, 9.7823) -> (99.6072, -3.2177)
  arc A324 (100.1072, -8.7677) -> (99.6072, -9.2677) centre (100.1072, -9.2677) ccw
  arc A325 (-57.8428, -9.2677) -> (-58.3428, -8.7677) centre (-58.3428, -9.2677) ccw
  arc A326 (-34.0303, -66.4177) -> (-34.5303, -65.9177) centre (-34.5303, -66.4177) ccw
  arc A327 (-88.5116, -98.4677) -> (-88.0116, -98.9677) centre (-88.0116, -98.4677) ccw
  arc A328 (123.9197, -65.9177) -> (123.4197, -66.4177) centre (123.9197, -66.4177) ccw
  line L340 (75.5072, -9.2677) -> (75.5072, -22.2677)
  line L341 (38.1947, -46.8677) -> (51.1947, -46.8677)
  arc A329 (176.3072, -65.9177) -> (175.8072, -66.4177) centre (176.3072, -66.4177) ccw
  line L342 (-88.0116, -84.9677) -> (-75.0116, -84.9677)
  line L343 (-40.8866, -85.4677) -> (-40.8866, -98.4677)
  line L344 (118.3697, -66.4177) -> (118.3697, -79.4177)
  arc A330 (151.2072, -3.7177) -> (151.7072, -3.2177) centre (151.2072, -3.2177) ccw
  arc A331 (22.6197, -79.9177) -> (23.1197, -79.4177) centre (22.6197, -79.4177) ccw
  arc A332 (-80.4246, -67.4177) -> (-80.9246, -66.9177) centre (-80.9246, -67.4177) ccw
  line L345 (18.3572, -9.2677) -> (18.3572, -22.2677)
  line L346 (-26.8866, -85.4677) -> (-26.8866, -98.4677)
  arc A333 (155.4629, -62.3677) -> (155.9629, -62.8677) centre (155.9629, -62.3677) ccw
  arc A334 (119.1572, -8.7677) -> (118.6572, -9.2677) centre (119.1572, -9.2677) ccw
  arc A335 (-39.2928, -3.7177) -> (-38.7928, -3.2177) centre (-39.2928, -3.2177) ccw
  line L347 (31.0509, -98.9677) -> (44.0509, -98.9677)
  line L348 (-64.9866, -66.4177) -> (-64.9866, -79.4177)
  line L349 (-87.4246, -67.4177) -> (-87.4246, -81.4177)
  arc A336 (17.8572, -22.7677) -> (18.3572, -22.2677) centre (17.8572, -22.2677) ccw
  arc A337 (-83.7491, -60.3677) -> (-83.2491, -60.8677) centre (-83.2491, -60.3677) ccw
  arc A338 (108.3447, -60.8677) -> (108.8447, -60.3677) centre (108.3447, -60.3677) ccw
  line L350 (176.3072, -65.9177) -> (189.3072, -65.9177)
  line L351 (151.7072, 9.7823) -> (151.7072, -3.2177)
  line L352 (-15.9491, -86.4677) -> (-15.9491, -100.4677)
  arc A339 (-52.2928, -8.7677) -> (-52.7928, -9.2677) centre (-52.2928, -9.2677) ccw
  line L353 (-15.4491, -100.9677) -> (-9.4491, -100.9677)
  line L354 (44.5509, -85.4677) -> (44.5509, -98.4677)
  arc A340 (57.2447, -46.8677) -> (56.7447, -47.3677) centre (57.2447, -47.3677) ccw
  arc A341 (85.3197, -79.4177) -> (85.8197, -79.9177) centre (85.8197, -79.4177) ccw
  line L355 (-48.0303, -66.4177) -> (-48.0303, -79.4177)
  line L356 (80.5572, -9.2677) -> (80.5572, -22.2677)
  arc A342 (-15.4803, -79.9177) -> (-14.9803, -79.4177) centre (-15.4803, -79.4177) ccw
  line L357 (56.4572, -9.2677) -> (56.4572, -22.2677)
  line L358 (138.2072, 10.2823) -> (151.2072, 10.2823)
  arc A343 (-74.5116, -85.4677) -> (-75.0116, -84.9677) centre (-75.0116, -85.4677) ccw
  line L359 (156.7572, 9.7823) -> (156.7572, -3.2177)
  line L360 (47.2197, -66.4177) -> (47.2197, -79.4177)
  arc A344 (9.1197, -79.4177) -> (9.6197, -79.9177) centre (9.6197, -79.4177) ccw
  arc A345 (44.0509, -98.9677) -> (44.5509, -98.4677) centre (44.0509, -98.4677) ccw
  line L361 (-50.6991, -85.4677) -> (-50.6991, -98.4677)